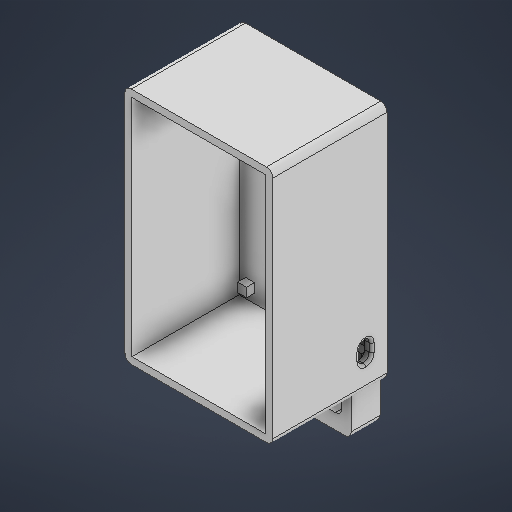
# Autodesk Inventor part: Part1
Saved by Autodesk Inventor 2026.3 (Build 303398000, 398)
## iProperties
Created: 2026-09-22
Part Number: Part1
Material: Generic
Document SubType Name: Modeling
Designer: arbaz
Density: 1 g/cm^3
Appearance: Default
Author: arbaz
Autodesk Inventor part; units mm, degrees
ref_plane "YZ Plane" through (0, 0, 0) normal (1, 0, 0) x (0, 1, 0)
ref_plane "XZ Plane" through (0, 0, 0) normal (0, 1, 0) x (-1, 0, 0)
ref_plane "XY Plane" through (0, 0, 0) normal (0, 0, 1) x (1, 0, 0)
sketch "Sketch1" plane through (0, 0, 0) normal (0, 0, 1) x (1, 0, 0)
  line L0 (0, 0) -> (70, 0)
  line L1 (70, 0) -> (70, 115)
  line L2 (70, 115) -> (0, 115)
  line L3 (0, 115) -> (0, 0)
  dimension "d0" = 70
  dimension "d1" = 115
  constraints: 8 end point, 2 parallel, 1 horizontal, 1 perpendicular
  measures "d0" distance of L2.end L1.end
  measures "d1" distance of L1.end L0.end
extrude "Extrusion1" add sketch "Sketch1" along normal blind 55
shell "Shell1" thickness 3.5 both sides yes removed faces 1 at (46.6667, 38.3333, 55)
sketch "Sketch2" plane through (1.75, 113.25, 1.75) normal (0, 0, 1) x (1, 0, 0)
  line L0 (3.175, -102.4355) -> (7.675, -102.4355)
  line L1 (7.675, -102.4355) -> (7.675, -106.9355)
  line L2 (7.675, -106.9355) -> (3.175, -106.9355)
  line L3 (3.175, -106.9355) -> (3.175, -102.4355)
  line L4 (60.325, -102.4355) -> (64.825, -102.4355)
  line L5 (64.825, -102.4355) -> (64.825, -106.9355)
  line L6 (64.825, -106.9355) -> (60.325, -106.9355)
  line L7 (60.325, -106.9355) -> (60.325, -102.4355)
  line L8 (3.175, -43.1855) -> (7.675, -43.1855)
  line L9 (7.675, -43.1855) -> (7.675, -47.6855)
  line L10 (7.675, -47.6855) -> (3.175, -47.6855)
  line L11 (3.175, -47.6855) -> (3.175, -43.1855)
  line L12 (3.175, -43.1855) -> (7.675, -47.6855) construction
  line L13 (7.675, -43.1855) -> (3.175, -47.6855) construction
  line L14 (60.325, -43.1855) -> (64.825, -43.1855)
  line L15 (64.825, -43.1855) -> (64.825, -47.6855)
  line L16 (64.825, -47.6855) -> (60.325, -47.6855)
  line L17 (60.325, -47.6855) -> (60.325, -43.1855)
  line L18 (60.325, -43.1855) -> (64.825, -47.6855) construction
  line L19 (64.825, -43.1855) -> (60.325, -47.6855) construction
  point P0 (-1.75, -113.25)
  dimension "d5" = 4.5
  dimension "d6" = 4.5
  dimension "d7" = 4.5
  dimension "d8" = 4.5
  dimension "d10" = 4.5
  dimension "d11" = 4.5
  dimension "d12" = 4.5
  dimension "d13" = 4.5
  constraints: 40 end point, 8 parallel, 4 horizontal, 4 perpendicular
  measures "d5" distance of L1.end L2.end
  measures "d6" distance of L0.end L1.end
  measures "d7" distance of L6.start L6.end
  measures "d8" distance of L5.start L6.start
  measures "d10" distance of L9.end L10.end
  measures "d11" distance of L8.end L9.end
  measures "d12" distance of L16.start L16.end
  measures "d13" distance of L14.end L16.start
extrude "Extrusion2" add sketch "Sketch2" along normal blind 4
sketch "Sketch4" plane through (71.75, -1.75, -1.75) normal (1, 0, 0) x (0, 0, -1)
  line L0 (-10.525, 12.077) -> (-10.875, 12.077)
  line L1 (-7.7, 15.252) -> (-7.7, 19.402)
  line L2 (-10.875, 22.577) -> (-10.525, 22.577)
  line L3 (-13.7, 19.402) -> (-13.7, 15.252)
  arc A0 (-13.7, 15.252) -> (-10.525, 12.077) centre (-10.525, 15.252) ccw
  arc A1 (-10.875, 12.077) -> (-7.7, 15.252) centre (-10.875, 15.252) ccw
  arc A2 (-10.525, 22.577) -> (-13.7, 19.402) centre (-10.525, 19.402) ccw
  arc A3 (-7.7, 19.402) -> (-10.875, 22.577) centre (-10.875, 19.402) ccw
  point P0 (-1.75, 1.75)
  point P1 (-13.7, 12.077)
  point P2 (-7.7, 22.577)
  point P3 (-7.7, 12.077)
  point P4 (-13.7, 22.577)
  point P5 (-10.7, 22.5722)
  point P6 (-10.7, 12.0819)
  dimension "d20" = 6
  dimension "d21" = 10.5
  dimension "d28" = 3.175
  constraints: 8 end point, 8 point on circle, 8 point on line, 8 tangent, 4 centre point, 3 equal radius, 2 parallel, 1 horizontal, 1 perpendicular
  measures "d20" distance of point (-13.7, 22.577) point (-7.7, 22.577)
  measures "d21" distance of point (-7.7, 22.577) point (-7.7, 12.077)
  measures "d28" radius of A0
extrude "Extrusion4" cut sketch "Sketch4" against normal blind 4 contours A0 L3 A2 A3 L1 A1
fillet "Fillet3" radius 3.175 1 edges at (71.75, -1.75, 26.625)
fillet "Fillet4" radius 3.175 3 edges at (-1.75, -1.75, 26.625) (-1.75, 116.75, 26.625) (71.75, 116.75, 26.625)
fillet "Fillet5" radius 1.27 6 edges at (71.75, 11.3197, 11.0811) (71.75, 15.577, 11.95) (71.75, 19.8343, 11.0811) (71.75, 15.577, 5.95) (71.75, 19.8343, 6.8189) (71.75, 11.3197, 6.8189)
sketch "Sketch5" plane through (68.575, -1.75, -1.75) normal (0, -1, 0) x (1, 0, 0)
  line L0 (-0.325, 3.5) -> (-0.325, 56.75) projected
  line L1 (-66.675, 14.2875) -> (-0.325, 14.2875)
  line L2 (-0.325, 14.2875) -> (-0.325, 0)
  line L3 (-0.325, 0) -> (-66.675, 0)
  line L4 (-66.675, 0) -> (-66.675, 14.2875)
  point P0 (-68.575, 1.75)
  constraints: 8 end point, 2 parallel, 1 horizontal, 1 perpendicular, 1 point on line
extrude "Extrusion5" add sketch "Sketch5" along normal blind 20
sketch "Sketch6" plane through (0, 0, -1.75) normal (0, 0, -1) x (-1, 0, 0)
  line L0 (-1.425, -1.75) -> (-68.575, -1.75) projected
  line L1 (-6.35, -14.25) -> (-63.5, -14.25)
  line L2 (-63.5, -14.25) -> (-63.5, -1.75)
  line L3 (-63.5, -1.75) -> (-6.35, -1.75)
  line L4 (-6.35, -1.75) -> (-6.35, -14.25)
  point P0 (0, 0)
  point P1 (-6.35, -1.75)
  constraints: 8 end point, 2 parallel, 1 horizontal, 1 perpendicular, 1 point on line
extrude "Extrusion6" cut sketch "Sketch6" against normal blind 25
fillet "Fillet6" radius 3.175 4 edges at (68.25, -21.75, 5.3938) (1.9, -21.75, 5.3937) (6.35, -14.25, 5.3938) (63.5, -14.25, 5.3938)
body "Solid1"
